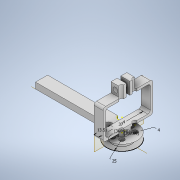
# Autodesk Inventor part: Marker holder
Saved by Autodesk Inventor 2022 (Build 260153000, 153)
## iProperties
Created: 2022-07-18
Part Number: Marker holder
Material: Generic
Document SubType Name: Modeling
Designer: biom
Density: 1 g/cm^3
Appearance: Default
Author: biom
Autodesk Inventor part; units mm, degrees
ref_plane "YZ Plane" through (0, 0, 0) normal (1, 0, 0) x (0, 1, 0)
ref_plane "XZ Plane" through (0, 0, 0) normal (0, 1, 0) x (-1, 0, 0)
ref_plane "XY Plane" through (0, 0, 0) normal (0, 0, 1) x (1, 0, 0)
sketch "Sketch1" plane through (0, 0, 0) normal (0, 1, 0) x (-1, 0, 0)
  circle A0 centre (0, 0) radius 12.5
  line L0 (0, 0) -> (7.75, 0) construction
  circle A1 centre (5.4801, -5.4801) radius 2
  circle A2 centre (-5.4801, -5.4801) radius 2
  circle A3 centre (-5.4801, 5.4801) radius 2
  circle A4 centre (5.4801, 5.4801) radius 2
  circle A5 centre (0, -7.75) radius 2
  circle A6 centre (0, 7.75) radius 2
  dimension "d0" = 25
  dimension "d3" = 4
  dimension "d6" = 360
  dimension "d8" = 4
  dimension "d11" = 360
  constraints: 7 centre point, 3 coincident, 2 end point, 1 horizontal, 16 other
  measures "d0" diameter of A0
  measures "d3" diameter of A1
  measures "d8" diameter of A5
extrude "Extrusion1" add sketch "Sketch1" along normal blind 5
sketch "Sketch2" plane through (0, 5, 0) normal (0, 1, 0) x (1, 0, 0)
  line L0 (4.991, -3.5408) -> (4.991, 3.5408)
  line L1 (-66.4503, 5) -> (-66.4503, -5)
  line L2 (4.991, -4.9385) -> (14.991, -4.9385) construction
  line L3 (-82.7386, 0) -> (31.2793, 0) projected
  arc A0 (-3.5548, -4.9385) -> (-7.4216, -5) centre (-5.4801, -5.4801) ccw
  line L4 (-66.4503, -5) -> (-7.4216, -5)
  line L5 (-3.5548, -4.9385) -> (3.5548, -4.9385)
  circle A1 centre (-5.4801, 5.4801) radius 2 projected
  arc A2 (-7.4216, 5) -> (-3.5497, 4.9571) centre (-5.4801, 5.4801) ccw
  line L6 (3.5497, 4.9571) -> (-3.5497, 4.9571)
  line L7 (-7.4216, 5) -> (-66.4503, 5)
  arc A3 (4.991, -3.5408) -> (3.5548, -4.9385) centre (5.4801, -5.4801) ccw
  circle A4 centre (5.4801, 5.4801) radius 2 projected
  arc A5 (3.5497, 4.9571) -> (4.991, 3.5408) centre (5.4801, 5.4801) ccw
  dimension "d24" = 10
  dimension "d25" = 90
  dimension "d26" = 70
  dimension "d27" = 4
  dimension "d28" = 4
  dimension "d29" = 4
  dimension "d30" = 4
  constraints: 14 end point, 8 point on circle, 7 parallel, 4 centre point, 4 coincident, 2 perpendicular, 1 horizontal, 1 vertical
  measures "d24" distance of L2.start L6.start
  measures "d25" angle of L2 L0
  measures "d26" distance of L1.start L6.start
  measures "d27" diameter of A0
  measures "d28" diameter of A2
  measures "d29" diameter of A3
  measures "d30" diameter of A5
extrude "Extrusion2" add sketch "Sketch2" along normal blind 5 contours A3 L5 A0 L4 L1 L3 L0 | L3 L1 L7 A1 L6 A4 L0
sketch "Sketch4" plane through (0, 10, 0) normal (0, 1, 0) x (1, 0, 0)
  line L0 (-3.5548, -4.9385) -> (3.5548, -4.9385) projected
  line L1 (-3.5548, -4.9385) -> (3.5548, -4.9385)
  line L2 (3.5497, 4.9571) -> (-3.5497, 4.9571) projected
  line L3 (-3.5497, 4.9571) -> (3.5497, 4.9571)
  line L4 (-4.4956, -10.2074) -> (2.6201, -10.2074)
  point P0 (0, 0)
  constraints: 6 end point, 3 horizontal
sketch "Sketch8" plane through (0, 5, 0) normal (0, 1, 0) x (1, 0, 0)
  circle A0 centre (-5.4801, 5.4801) radius 2 projected
  circle A1 centre (-5.4801, 5.4801) radius 3
  circle A2 centre (-5.4801, -5.4801) radius 2 projected
  circle A3 centre (-5.4801, -5.4801) radius 3
  circle A4 centre (5.4801, 5.4801) radius 2 projected
  circle A5 centre (5.4801, 5.4801) radius 3
  arc A6 (3.5548, -4.9385) -> (4.991, -3.5408) centre (5.4801, -5.4801) ccw projected
  circle A7 centre (5.4801, -5.4801) radius 3
  point P0 (0, 0)
  dimension "d50" = 6
  dimension "d51" = 6
  dimension "d52" = 6
  dimension "d53" = 6
  constraints: 4 centre point, 4 coincident
  measures "d50" diameter of A1
  measures "d51" diameter of A3
  measures "d52" diameter of A5
  measures "d53" diameter of A7
extrude "Extrusion6" cut sketch "Sketch8" along normal blind 39.25 contours A0 | A1 | A2 | A3 | A4 | A5 | A7
sketch "Sketch30" plane through (0, 10, 0) normal (0, 1, 0) x (1, 0, 0)
  line L0 (-2.5294, -4.9385) -> (2.5294, -4.9385) projected
  arc A0 (-8.4414, 5) -> (-2.526, 4.9571) centre (-5.4801, 5.4801) ccw projected
  line L1 (-2.5294, -18.4485) -> (-2.5294, 18.5515)
  arc A1 (4.991, -2.5202) -> (2.5294, -4.9385) centre (5.4801, -5.4801) ccw projected
  arc A2 (2.526, 4.9571) -> (4.991, 2.5202) centre (5.4801, 5.4801) ccw projected
  point P0 (0, 0)
  dimension "d90" = 13.51
  dimension "d91" = 37
  constraints: 2 end point
  measures "d90" distance of L0.start L1.start
  measures "d91" distance of L1.start L1.end
sketch "Sketch31" plane through (4.991, 5, 2.5202) normal (1, 0, 0) x (0, 0, -1)
  point P0 (2.5202, -5)
ref_plane "Work Plane4" through (-2.5294, 10, 18.4485) normal (1, 0, 0) x (0, 0, -1)
sketch "Sketch41" plane through (-2.5294, 10, 18.4485) normal (1, 0, 0) x (0, 0, -1)
  line L0 (0, 0) -> (-2, 0)
  line L1 (-2, 0) -> (39, 0)
  line L2 (15.9283, 0) -> (20.9687, 0) projected
  line L3 (39, 0) -> (39, 25)
  line L4 (-2, 25) -> (-2, 0)
  line L5 (18.5, 1.9993) -> (0, 1.9993)
  line L6 (18.5, 1.9993) -> (37, 1.9993)
  line L7 (0, 1.9993) -> (37, 1.9993)
  line L8 (37, 23) -> (37, 1.9993)
  line L9 (0, 12.5) -> (0, 23)
  line L10 (0, 23) -> (0, 1.9993)
  line L11 (17, 23) -> (17, 33)
  line L12 (17, 33) -> (12, 33)
  line L13 (12, 33) -> (12, 25)
  line L14 (20, 23) -> (20, 33)
  line L15 (20, 33) -> (25, 33)
  line L16 (25, 33) -> (25, 25)
  line L17 (25, 25) -> (39, 25)
  line L18 (39, 25) -> (39, 0)
  line L19 (39, 0) -> (-2, 0)
  line L20 (30.9485, -10) -> (5.9485, -10) projected
  line L21 (-2, 0) -> (-2, 25)
  line L22 (-2, 25) -> (12, 25)
  line L23 (12, 33) -> (17, 33)
  line L24 (17, 33) -> (17, 23)
  line L25 (17, 23) -> (0, 23)
  line L26 (0, 23) -> (0, 1.9993)
  line L27 (37, 1.9993) -> (0, 1.9993)
  line L28 (30.9485, -5) -> (5.9485, -5) projected
  line L29 (37, 1.9993) -> (37, 23)
  line L30 (37, 23) -> (20, 23)
  line L31 (20, 23) -> (20, 33)
  line L32 (25, 33) -> (25, 25)
  point P0 (18.4485, -10)
  point P1 (13.4485, -5)
  point P2 (23.4485, -5)
  point P3 (0, 12.5)
  dimension "d129" = 2
  dimension "d130" = 41
  dimension "d131" = 25
  dimension "d132" = 41
  dimension "d138" = 3
  dimension "d139" = 10
  dimension "d140" = 5
  dimension "d141" = 5
  constraints: 60 end point, 7 collinear, 4 parallel, 3 point on line, 1 horizontal, 1 perpendicular, 1 vertical
  measures "d129" distance of L0.start L0.end
  measures "d130" distance of L0.end L1.end
  measures "d131" distance of L1.end L3.end
  measures "d132" distance of L3.end L4.start
  measures "d138" distance of L14.start L11.start
  measures "d139" distance of L11.start L11.end
  measures "d140" distance of L11.end L12.end
  measures "d141" distance of L14.end L15.end
extrude "Extrusion14" add sketch "Sketch41" along normal up to surface (7.5204 mm away)
sketch "Sketch42" plane through (-2.5294, 35, 6.4485) normal (0, 0, 1) x (1, 0, 0)
  line L0 (0, 0) -> (0, 8) projected
  line L1 (7.5204, -2) -> (7.5204, 8) projected
  line L2 (0, 8) -> (7.5204, 8) projected
  circle A0 centre (3.7602, 3.8975) radius 2
  point P0 (2.5294, -35)
  dimension "d144" = 4
  constraints: 1 centre point
  measures "d144" diameter of A0
extrude "Extrusion15" cut sketch "Sketch42" against normal through all
fillet "Fillet3" radius 2 8 edges at (1.2308, 11.9993, 18.4485) (1.2308, 10, 20.4485) (1.2308, 10, -20.5515) (1.2308, 35, -20.5515) (1.2308, 33, -18.5515) (1.2308, 11.9993, -18.5515) (1.2308, 33, 18.4485) (1.2308, 35, 20.4485)
extrude "Extrusion17" cut sketch "Sketch1" along normal through all contours A2 | A3
body "Solid1"
